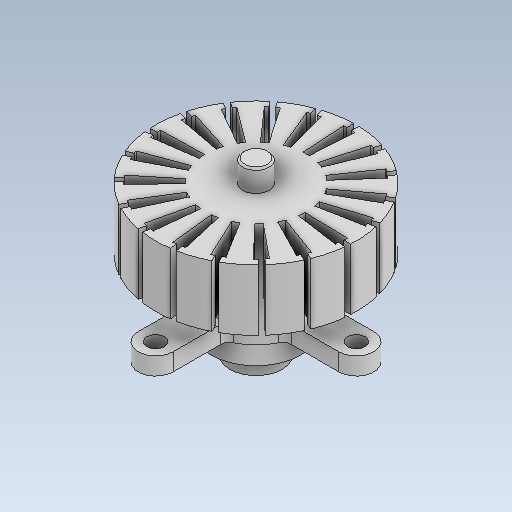
# Autodesk Inventor part: mot_27_2
Saved by Autodesk Inventor 2023 (Build 270158000, 158)
## iProperties
Created: 2020-12-02
Part Number: mot_27_2
Material: Generic
Document SubType Name: Modeling
Designer: Shuang Peng
Density: 1 g/cm^3
Appearance: Default
Author: Shuang Peng
Autodesk Inventor part; units mm, degrees
ref_plane "YZ Plane" through (0, 0, 0) normal (1, 0, 0) x (0, 1, 0)
ref_plane "XZ Plane" through (0, 0, 0) normal (0, 1, 0) x (-1, 0, 0)
sketch "Sketch1" plane through (0, 0, 0) normal (0, 1, 0) x (-1, 0, 0)
  circle A0 centre (0, 0) radius 5.75
  dimension "d0" = 11.5
  constraints: 1 centre point, 1 coincident
  measures "d0" diameter of A0
extrude "Extrusion1" add sketch "Sketch1" along normal blind 5
sketch "Sketch2" plane through (0, 0, 0) normal (0, -1, 0) x (1, 0, 0)
  circle A0 centre (0, 0) radius 5.15
  dimension "d3" = 10.3
  constraints: 1 centre point, 1 coincident
  measures "d3" diameter of A0
extrude "Extrusion2" add sketch "Sketch2" along normal blind 2.5
sketch "Sketch3" plane through (0, -2.5, 0) normal (0, -1, 0) x (1, 0, 0)
  circle A0 centre (0, 0) radius 5.15 projected
  circle A1 centre (0, 0) radius 3.8
  dimension "d6" = 1.35
  constraints: 1 centre point, 1 coincident
  measures "d6" radial gap between concentric circles of A0 A1
extrude "Extrusion3" cut sketch "Sketch3" against normal blind 1.7 contours A1
sketch "Sketch4" plane through (0, 0, 0) normal (0, -1, 0) x (1, 0, 0)
  line L0 (0, 0) -> (0, 11.5)
  line L1 (0, 11.5) -> (0, -11.5) construction
  line L2 (-2, 11.5) -> (-2, -11.5)
  line L3 (2, -11.5) -> (2, 11.5)
  arc A0 (2, 11.5) -> (-2, 11.5) centre (0, 11.5) ccw
  arc A1 (-2, -11.5) -> (2, -11.5) centre (0, -11.5) ccw
  line L4 (0, 0) -> (11.5, 0)
  line L5 (11.5, 0) -> (-11.5, 0) construction
  line L6 (11.5, 2) -> (-11.5, 2)
  line L7 (-11.5, -2) -> (11.5, -2)
  arc A2 (11.5, -2) -> (11.5, 2) centre (11.5, 0) ccw
  arc A3 (-11.5, 2) -> (-11.5, -2) centre (-11.5, 0) ccw
  circle A4 centre (0, 0) radius 5.75 projected
  point P0 (-2, 5.391)
  point P1 (2, 5.391)
  point P2 (-5.391, -2)
  point P3 (-5.391, 2)
  point P4 (2, -5.391)
  point P5 (-2, -5.391)
  point P6 (5.391, 2)
  point P7 (5.391, -2)
  dimension "d9" = 11.5
  dimension "d10" = 23
  dimension "d11" = 4
  dimension "d12" = 11.5
  dimension "d13" = 23
  dimension "d14" = 4
  constraints: 20 end point, 8 point on circle, 8 tangent, 4 centre point, 2 horizontal, 2 midpoint, 2 parallel, 1 point on line, 1 vertical
  measures "d9" distance of L0.start L0.end
  measures "d10" distance of L0.end L1.end
  measures "d11" diameter of A1
  measures "d12" distance of L4.start L4.end
  measures "d13" distance of L4.end L5.end
  measures "d14" diameter of A3
extrude "Extrusion4" add sketch "Sketch4" against normal blind 2 contours A4 L2 A0 L3 | A4 L6 A2 L7 | A4 L7 A3 L6 | L3 A1 L2 A4
sketch "Sketch5" plane through (0, 0, 0) normal (0, -1, 0) x (1, 0, 0)
  circle A0 centre (0, 0) radius 5.15 projected
  line L0 (-5.391, 2) -> (-11.5, 2) projected
  arc A1 (-11.5, 2) -> (-11.5, -2) centre (-11.5, 0) ccw projected
  line L1 (-11.5, -2) -> (-5.391, -2) projected
  arc A2 (-5.391, -2) -> (-2, -5.391) centre (0, 0) ccw projected
  line L2 (-2, -5.391) -> (-2, -11.5) projected
  arc A3 (-2, -11.5) -> (2, -11.5) centre (0, -11.5) ccw projected
  line L3 (2, -11.5) -> (2, -5.391) projected
  arc A4 (2, -5.391) -> (5.391, -2) centre (0, 0) ccw projected
  line L4 (5.391, -2) -> (11.5, -2) projected
  arc A5 (11.5, -2) -> (11.5, 2) centre (11.5, 0) ccw projected
  line L5 (11.5, 2) -> (5.391, 2) projected
  arc A6 (5.391, 2) -> (2, 5.391) centre (0, 0) ccw projected
  line L6 (2, 5.391) -> (2, 11.5) projected
  arc A7 (2, 11.5) -> (-2, 11.5) centre (0, 11.5) ccw projected
  line L7 (-2, 11.5) -> (-2, 5.391) projected
  arc A8 (-2, 5.391) -> (-5.391, 2) centre (0, 0) ccw projected
hole "Hole1" at (11.5, 0, 0) at (0, 0, -11.5) at (-11.5, 0, 0) at (0, 0, 11.5) direction (0, 1, 0) diameter 2 depth 5
fillet "Fillet1" radius 1 8 edges at (5.391, 1, -2) (2, 1, -5.391) (5.391, 1, 2) (2, 1, 5.391) (-2, 1, 5.391) (-5.391, 1, 2) (-5.391, 1, -2) (-2, 1, -5.391)
sketch "Sketch6" plane through (0, -0.8, 0) normal (0, -1, 0) x (1, 0, 0)
  circle A0 centre (0, 0) radius 3
  dimension "d25" = 6
  constraints: 1 centre point, 1 coincident
  measures "d25" diameter of A0
extrude "Extrusion5" add sketch "Sketch6" along normal blind 4.2
sketch "Sketch7" plane through (0, 5, 0) normal (0, 1, 0) x (1, 0, 0)
  circle A0 centre (0, 0) radius 5.75 projected
  circle A1 centre (0, 0) radius 11.5
  line L0 (0, 0) -> (1.2021, -11.437)
  line L1 (0, 0) -> (0, -11.5)
  line L2 (0, 0) -> (-1.2021, -11.437)
  circle A2 centre (0, 0) radius 10.7
  line L3 (0, 0) -> (1.6005, -11.3881)
  line L4 (0, 0) -> (-1.6005, -11.3881)
  point P0 (0.601, -5.7185)
  point P1 (-0.601, -5.7185)
  point P2 (-1.1185, -10.6414)
  point P3 (-1.4892, -10.5959)
  point P4 (1.4892, -10.5959)
  point P5 (1.1185, -10.6414)
  dimension "d28" = 23
  dimension "d29" = 6
  dimension "d30" = 6
  dimension "d31" = 0.8
  dimension "d32" = 2
  dimension "d33" = 2
  constraints: 10 end point, 5 point on circle, 2 centre point, 2 coincident, 1 vertical
  measures "d28" diameter of A1
  measures "d29" angle of L1 L2
  measures "d30" angle of L1 L0
  measures "d31" radial gap between concentric circles of A1 A2
  measures "d32" angle of L2 L4
  measures "d33" angle of L0 L3
extrude "Extrusion6" add sketch "Sketch7" along normal blind 7 contours A0 L3 L4 | L4 L2 A0 | A0 L0 L3 | L2 L1 A0 | A0 L1 A2 L2 | L0 A0 L1 | A2 L2 A1 L4 | L0 A2 L1 A0 | L3 A1 L0 A2 | A2 L1 A1 L2 | L0 A1 L1 A2
pattern_circular "Circular Pattern1" count 19 over 360 about axis through (0, 0, 0) along (0, 1, 0) of "Extrusion6"
sketch "Sketch8" plane through (0, 12, 0) normal (0, 1, 0) x (1, 0, 0)
  circle A0 centre (0, 0) radius 1.5
  dimension "d39" = 3
  constraints: 1 centre point, 1 coincident
  measures "d39" diameter of A0
ref_plane "Work Plane1" through (-17.4612, 14.5, -17.4612) normal (0, 1, 0) x (-0.5689786, 0, 0.8223523)
extrude "Extrusion7" add sketch "Sketch8" along normal up to surface (2.5 mm away)
chamfer "Chamfer1" distance 0.2 angle 45 1 edges at (-1.5, 14.5, 0)
body "Solid1"
